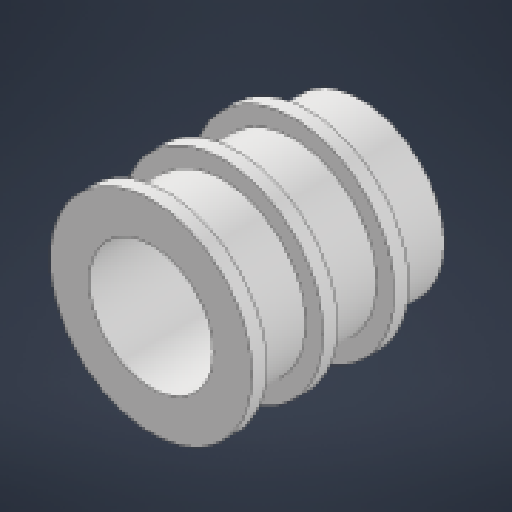
# Autodesk Inventor part: puleggia motore
Saved by Autodesk Inventor 2024.3 (Build 283343000, 343)
## iProperties
Created: 2025-08-22
Part Number: puleggia motore
Material: Generic
Document SubType Name: Modeling
Designer: giuseppe
Density: 1 g/cm^3
Appearance: Default
Author: giuseppe
Autodesk Inventor part; units mm, degrees
ref_plane "YZ Plane" through (0, 0, 0) normal (1, 0, 0) x (0, 1, 0)
ref_plane "XZ Plane" through (0, 0, 0) normal (0, 1, 0) x (-1, 0, 0)
ref_plane "XY Plane" through (0, 0, 0) normal (0, 0, 1) x (1, 0, 0)
sketch "Sketch1" plane through (0, 0, 0) normal (0, 0, 1) x (1, 0, 0)
  circle A0 centre (0, 0) radius 3.5
  circle A1 centre (0, 0) radius 0.8 construction
  circle A2 centre (0, 0) radius 1
  dimension "d0" = 7
  dimension "d1" = 2
  constraints: 2 centre point, 2 coincident, 1 concentric
  measures "d0" diameter of A0
  measures "d1" diameter of A2
extrude "Extrusion1" add sketch "Sketch1" along normal blind 1
sketch "Sketch2" plane through (0, 0, 0) normal (0, 0, -1) x (-1, 0, 0)
  circle A0 centre (0, 0) radius 4.7
  circle A1 centre (0, 0) radius 3.5 projected
  dimension "d4" = 1.2
  constraints: 1 centre point, 1 coincident
  measures "d4" radial gap between concentric circles of A0 A1
ref_plane "Work Plane1" through (-8.6503, -26.6, 11.8) normal (0, 0, 1) x (1, 0, 0)
extrude "Extrusion2" add sketch "Sketch2" against normal up to surface (11.8 mm away)
sketch "Sketch3" plane through (0, 0, 11.8) normal (0, 0, 1) x (1, 0, 0)
  circle A0 centre (0, 0) radius 5.7
  circle A1 centre (0, 0) radius 4.7 projected
  dimension "d7" = 1
  constraints: 1 centre point, 1 coincident
  measures "d7" radial gap between concentric circles of A0 A1
ref_plane "Work Plane2" through (-8.6503, -26.6, 11) normal (0, 0, -1) x (0, 1, 0)
extrude "Extrusion3" add sketch "Sketch3" against normal up to surface (0.8 mm away)
pattern_linear "Rectangular Pattern1" count 3 spacing 4 along (0, 0, -1) of "Extrusion3"
body "Solid1"
